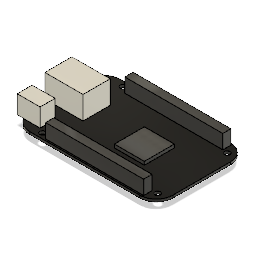
BeagleBoneBlack (Autodesk Fusion 360 design; units mm, degrees)
Autodesk Fusion 360 part; units mm, degrees
sketch "Sketch1" plane through (0, 0, 0) normal (0, 1, 0) x (1, 0, 0)
  line L0 (10, 0) -> (76.2, 0)
  line L1 (86.2, 10) -> (86.2, 44.61)
  line L2 (76.2, 54.61) -> (10, 54.61)
  line L3 (0, 44.61) -> (0, 10)
  circle A0 centre (14.6, 51.435) radius 1.6
  circle A1 centre (14.6, 3.175) radius 1.6
  circle A2 centre (80.64, 48.26) radius 1.6
  circle A3 centre (80.64, 6.35) radius 1.6
  arc A4 (0, 10) -> (10, 0) centre (10, 10) ccw
  arc A5 (10, 54.61) -> (0, 44.61) centre (10, 44.61) ccw
  arc A6 (86.2, 44.61) -> (76.2, 54.61) centre (76.2, 44.61) ccw
  arc A7 (76.2, 0) -> (86.2, 10) centre (76.2, 10) ccw
  dimension "d1" = 86.2
  dimension "d2" = 54.61
  dimension "d3" = 3.2
  dimension "d4" = 14.6
  dimension "d5" = 3.175
  dimension "d6" = 48.26
  dimension "d8" = 41.91
  dimension "d10" = 6.35
  dimension "d11" = 65.9
  dimension "d12" = 66.04
  dimension "d13" = 10
  dimension "d36" = 3.11
  measures "d1" distance of origin
  measures "d2" distance of origin
  measures "d3" diameter of A1
  measures "d4" distance of L3
  measures "d5" distance of L2
  measures "d8" distance of origin
  measures "d10" distance of L0
  measures "d12" distance of origin
  measures "d13" radius of A4
extrude "Extrude1" add sketch "Sketch1" along normal blind 1.6
sketch "Sketch2" plane through (0, 1.6, 0) normal (0, 1, 0) x (-1, 0, 0)
  circle A0 centre (-14.6, -3.175) radius 1.6
  circle A1 centre (-80.64, -6.35) radius 1.6
  circle A2 centre (-14.6, -51.435) radius 1.6
  circle A3 centre (-80.64, -48.26) radius 1.6
  arc A4 (-76.2, 0) -> (-86.2, -10) centre (-76.2, -10) ccw
  line L0 (-86.2, -10) -> (-86.2, -44.61)
  arc A5 (-86.2, -44.61) -> (-76.2, -54.61) centre (-76.2, -44.61) ccw
  line L1 (-76.2, -54.61) -> (-10, -54.61)
  arc A6 (-10, -54.61) -> (0, -44.61) centre (-10, -44.61) ccw
  line L2 (0, -44.61) -> (0, -10)
  arc A7 (0, -10) -> (-10, 0) centre (-10, -10) ccw
  line L3 (-10, 0) -> (-76.2, 0)
  line L4 (-18.553, -6) -> (-77.553, -6)
  line L5 (-77.553, -6) -> (-77.553, -1)
  line L6 (-77.553, -1) -> (-18.553, -1)
  line L7 (-18.553, -1) -> (-18.553, -6)
  line L8 (-18.553, -53.61) -> (-77.553, -53.61)
  line L9 (-77.553, -53.61) -> (-77.553, -48.61)
  line L10 (-77.553, -48.61) -> (-18.553, -48.61)
  line L11 (-18.553, -48.61) -> (-18.553, -53.61)
  dimension "d16" = 59
  dimension "d17" = 1
  dimension "d18" = 1
  dimension "d19" = 5
  measures "d16" distance of origin
  measures "d17" distance of L1 L8
  measures "d18" distance of L3 L6
extrude "Extrude2" add sketch "Sketch2" along normal blind 8.5 contours L4 L5 L6 L7 | L8 L9 L10 L11
sketch "Sketch3" plane through (0, 1.6, 0) normal (0, 1, 0) x (-1, 0, 0)
  line L0 (-18.553, -1) -> (-18.553, -6)
  line L1 (-18.553, -6) -> (-77.553, -6)
  line L2 (-77.553, -6) -> (-77.553, -1)
  line L3 (-77.553, -1) -> (-18.553, -1)
  line L4 (-18.553, -48.61) -> (-18.553, -53.61)
  line L5 (-18.553, -53.61) -> (-77.553, -53.61)
  line L6 (-77.553, -53.61) -> (-77.553, -48.61)
  line L7 (-77.553, -48.61) -> (-18.553, -48.61)
  circle A0 centre (-14.6, -3.175) radius 1.6
  circle A1 centre (-80.64, -6.35) radius 1.6
  circle A2 centre (-14.6, -51.435) radius 1.6
  circle A3 centre (-80.64, -48.26) radius 1.6
  arc A4 (-76.2, 0) -> (-86.2, -10) centre (-76.2, -10) ccw
  line L8 (-86.2, -10) -> (-86.2, -44.61)
  arc A5 (-86.2, -44.61) -> (-76.2, -54.61) centre (-76.2, -44.61) ccw
  line L9 (-76.2, -54.61) -> (-10, -54.61)
  arc A6 (-10, -54.61) -> (0, -44.61) centre (-10, -44.61) ccw
  line L10 (0, -44.61) -> (0, -10)
  arc A7 (0, -10) -> (-10, 0) centre (-10, -10) ccw
  line L11 (-10, 0) -> (-76.2, 0)
  line L12 (2.5, -37.91) -> (-20.5, -37.91)
  line L13 (-20.5, -37.91) -> (-20.5, -21.61)
  line L14 (-20.5, -21.61) -> (2.5, -21.61)
  line L15 (2.5, -21.61) -> (2.5, -37.91)
  dimension "d22" = 16.3
  dimension "d23" = 16.7
  dimension "d24" = 2.5
  measures "d23" distance of L9 L12
  measures "d24" distance of L10 L15
extrude "Extrude3" add sketch "Sketch3" along normal blind 13.8 contours L10 L12 L14 L15 | L10 L12 L13 L14
sketch "Sketch4" plane through (0, 1.6, 0) normal (0, 1, 0) x (-1, 0, 0)
  line L0 (-20.5, -21.61) -> (0, -21.61)
  line L1 (0, -21.61) -> (0, -10)
  arc A0 (0, -10) -> (-10, 0) centre (-10, -10) ccw
  line L2 (-10, 0) -> (-76.2, 0)
  arc A1 (-76.2, 0) -> (-86.2, -10) centre (-76.2, -10) ccw
  line L3 (-86.2, -10) -> (-86.2, -44.61)
  arc A2 (-86.2, -44.61) -> (-76.2, -54.61) centre (-76.2, -44.61) ccw
  line L4 (-76.2, -54.61) -> (-10, -54.61)
  arc A3 (-10, -54.61) -> (0, -44.61) centre (-10, -44.61) ccw
  line L5 (0, -44.61) -> (0, -37.91)
  line L6 (0, -37.91) -> (-20.5, -37.91)
  line L7 (-20.5, -37.91) -> (-20.5, -21.61)
  line L8 (-18.553, -1) -> (-18.553, -6)
  line L9 (-18.553, -6) -> (-77.553, -6)
  line L10 (-77.553, -6) -> (-77.553, -1)
  line L11 (-77.553, -1) -> (-18.553, -1)
  line L12 (-18.553, -48.61) -> (-18.553, -53.61)
  line L13 (-18.553, -53.61) -> (-77.553, -53.61)
  line L14 (-77.553, -53.61) -> (-77.553, -48.61)
  line L15 (-77.553, -48.61) -> (-18.553, -48.61)
  circle A4 centre (-14.6, -3.175) radius 1.6
  circle A5 centre (-80.64, -6.35) radius 1.6
  circle A6 centre (-14.6, -51.435) radius 1.6
  circle A7 centre (-80.64, -48.26) radius 1.6
  line L16 (2.5, -14) -> (-11.3258, -14)
  line L17 (-11.3258, -14) -> (-11.3258, -5)
  line L18 (-11.3258, -5) -> (2.5, -5)
  line L19 (2.5, -5) -> (2.5, -14)
  dimension "d27" = 9
  dimension "d28" = 5
  measures "d28" distance of L18
extrude "Extrude4" add sketch "Sketch4" along normal blind 11 contours L1 A0 L16 L17 L18 | L1 A0 L16 L18 L19
sketch "Sketch5" plane through (0, 0, 0) normal (0, -1, 0) x (1, 0, 0)
  circle A0 centre (14.6, -3.175) radius 1.6
  circle A1 centre (80.64, -6.35) radius 1.6
  circle A2 centre (14.6, -51.435) radius 1.6
  circle A3 centre (80.64, -48.26) radius 1.6
  arc A4 (86.2, -10) -> (76.2, 0) centre (76.2, -10) ccw
  line L0 (76.2, 0) -> (10, 0)
  arc A5 (10, 0) -> (0, -10) centre (10, -10) ccw
  line L1 (0, -10) -> (0, -44.61)
  arc A6 (0, -44.61) -> (10, -54.61) centre (10, -44.61) ccw
  line L2 (10, -54.61) -> (76.2, -54.61)
  arc A7 (76.2, -54.61) -> (86.2, -44.61) centre (76.2, -44.61) ccw
  line L3 (86.2, -44.61) -> (86.2, -10)
  line L4 (-0.5891, -40.4049) -> (7.6203, -40.4049)
  line L5 (7.6203, -40.4049) -> (7.6203, -46.4306)
  line L6 (7.6203, -46.4306) -> (-0.5891, -46.4306)
  line L7 (-0.5891, -46.4306) -> (-0.5891, -40.4049)
extrude "Extrude5" add sketch "Sketch5" along normal blind 3.9 contours L1 A6 L4 L5 L6 | L1 A6 L4 L6 L7
sketch "Sketch6" plane through (0, 1.6, 0) normal (0, 1, 0) x (-1, 0, 0)
  line L0 (-11.3258, -5) -> (-1.3397, -5)
  arc A0 (-1.3397, -5) -> (-10, 0) centre (-10, -10) ccw
  line L1 (-10, 0) -> (-76.2, 0)
  arc A1 (-76.2, 0) -> (-86.2, -10) centre (-76.2, -10) ccw
  line L2 (-86.2, -10) -> (-86.2, -44.61)
  arc A2 (-86.2, -44.61) -> (-76.2, -54.61) centre (-76.2, -44.61) ccw
  line L3 (-76.2, -54.61) -> (-10, -54.61)
  arc A3 (-10, -54.61) -> (0, -44.61) centre (-10, -44.61) ccw
  line L4 (0, -44.61) -> (0, -37.91)
  line L5 (0, -37.91) -> (-20.5, -37.91)
  line L6 (-20.5, -37.91) -> (-20.5, -21.61)
  line L7 (-20.5, -21.61) -> (0, -21.61)
  line L8 (0, -21.61) -> (0, -14)
  line L9 (0, -14) -> (-11.3258, -14)
  line L10 (-11.3258, -14) -> (-11.3258, -5)
  line L11 (-18.553, -1) -> (-18.553, -6)
  line L12 (-18.553, -6) -> (-77.553, -6)
  line L13 (-77.553, -6) -> (-77.553, -1)
  line L14 (-77.553, -1) -> (-18.553, -1)
  line L15 (-18.553, -48.61) -> (-18.553, -53.61)
  line L16 (-18.553, -53.61) -> (-77.553, -53.61)
  line L17 (-77.553, -53.61) -> (-77.553, -48.61)
  line L18 (-77.553, -48.61) -> (-18.553, -48.61)
  circle A4 centre (-14.6, -3.175) radius 1.6
  circle A5 centre (-80.64, -6.35) radius 1.6
  circle A6 centre (-14.6, -51.435) radius 1.6
  circle A7 centre (-80.64, -48.26) radius 1.6
  line L19 (-44, -35) -> (-62, -35)
  line L20 (-62, -35) -> (-62, -17)
  line L21 (-62, -17) -> (-44, -17)
  line L22 (-44, -17) -> (-44, -35)
  dimension "d33" = 18
  measures "d33" distance of origin
extrude "Extrude6" add sketch "Sketch6" along normal blind 2 contours L19 L20 L21 L22
